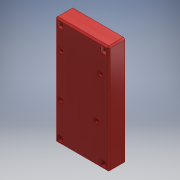
# Autodesk Inventor part: mangOH bottom
Saved by Autodesk Inventor 2017.3 (Build 213256000, 256)
## iProperties
Created: 2018-01-31
Part Number: mangOH bottom
Material: Generic
Document SubType Name: Modeling
Designer: michiel
Density: 1 g/cm^3
Appearance: Orange-Red
Author: michiel
Autodesk Inventor part; units mm, degrees
ref_plane "YZ Plane" through (0, 0, 0) normal (1, 0, 0) x (0, 1, 0)
ref_plane "XZ Plane" through (0, 0, 0) normal (0, 1, 0) x (-1, 0, 0)
ref_plane "XY Plane" through (0, 0, 0) normal (0, 0, 1) x (1, 0, 0)
sketch "Sketch1" plane through (0, 0, 0) normal (0, 1, 0) x (-1, 0, 0)
  line L0 (0, 0) -> (73, 0)
  line L1 (73, 0) -> (73, -148)
  line L2 (73, -148) -> (0, -148)
  line L3 (0, -148) -> (0, 0)
  dimension "d0" = 73
  dimension "d1" = 148
  constraints: 8 end point, 2 parallel, 1 horizontal, 1 perpendicular
  measures "d0" distance of L1.end L2.end
  measures "d1" distance of L0.end L1.end
extrude "Extrusion1" add sketch "Sketch1" against normal blind 4
sketch "Sketch2" plane through (0, 0, 0) normal (0, 1, 0) x (1, 0, 0)
  line L0 (-73, 148) -> (0, 148) projected
  line L1 (0, 148) -> (0, 0) projected
  line L2 (0, 148) -> (0, 0)
  line L3 (0, 0) -> (-73, 0) projected
  line L4 (0, 0) -> (-73, 0)
  line L5 (-73, 0) -> (-73, 148)
  line L6 (0, 148) -> (0, 144) construction
  line L7 (0, 148) -> (0, 0) construction
  line L8 (0, 144) -> (-4, 144) construction
  line L9 (-4, 144) -> (-69, 144)
  line L10 (-69, 144) -> (-69, 4)
  line L11 (-69, 4) -> (-4, 4)
  line L12 (-4, 4) -> (-4, 144)
  dimension "d4" = 4
  dimension "d5" = 4
  dimension "d6" = 90
  dimension "d7" = 65
  dimension "d8" = 140
  constraints: 18 end point, 3 perpendicular, 2 collinear, 2 horizontal, 1 point on line, 1 vertical
  measures "d4" distance of L0.end L6.end
  measures "d5" distance of L6.end L8.end
  measures "d6" angle of L6 L8
  measures "d7" distance of L8.end L9.end
  measures "d8" distance of L9.end L10.end
extrude "Extrusion2" add sketch "Sketch2" along normal blind 18
sketch "Sketch4" plane through (0, 0, 0) normal (0, 1, 0) x (1, 0, 0)
  line L0 (-4, 4) -> (-4, 144) projected
  line L1 (-4, 4) -> (-10, 4)
  line L2 (-10, 4) -> (-10, 10)
  line L3 (-10, 10) -> (-4, 10)
  line L4 (-4, 10) -> (-4, 4)
  point P0 (0, 0)
  dimension "d17" = 6
  dimension "d18" = 6
  constraints: 8 end point, 2 parallel, 1 horizontal, 1 perpendicular
  measures "d17" distance of L2.end L3.end
  measures "d18" distance of L1.end L2.end
extrude "Extrusion4" add sketch "Sketch4" along normal blind 15
sketch "Sketch9" plane through (0, -4, 0) normal (0, -1, 0) x (1, 0, 0)
  line L0 (0, 0) -> (0, -148) construction
  line L1 (0, 0) -> (-7, 0) construction
  line L2 (0, 0) -> (-73, 0) construction
  line L3 (-7, 0) -> (-7, -7) construction
  circle A0 centre (-7, -7) radius 2.05
  dimension "d60" = 7
  dimension "d61" = 7
  dimension "d62" = 4.1
  constraints: 4 end point, 1 centre point, 1 coincident, 1 perpendicular, 1 point on line
  measures "d60" distance of L0.start L1.end
  measures "d61" distance of L1.end L3.end
  measures "d62" diameter of A0
extrude "Extrusion10" cut sketch "Sketch9" against normal blind 20
sketch "Sketch10" plane through (0, -4, 0) normal (0, -1, 0) x (1, 0, 0)
  circle A0 centre (-7, -7) radius 2.05 construction
  line L0 (-7, -7) -> (-7, 0) construction
  line L1 (0, 0) -> (-73, 0) construction
  line L2 (-7, -7) -> (-10.6, -7) construction
  line L3 (-7, -7) -> (-3.4, -7) construction
  line L4 (-7, -7) -> (-7, -10.875) construction
  line L5 (-7, -7) -> (-7, -3.125) construction
  line L6 (-7, -3.125) -> (-10.6, -3.125)
  line L7 (-10.6, -3.125) -> (-10.6, -10.875)
  line L8 (-10.6, -10.875) -> (-3.4, -10.875)
  line L9 (-3.4, -10.875) -> (-3.4, -3.125)
  line L10 (-3.4, -3.125) -> (-7, -3.125)
  dimension "d65" = 3.6
  dimension "d66" = 3.6
  dimension "d67" = 3.875
  dimension "d68" = 3.875
  dimension "d69" = 7.75
  dimension "d70" = 7.2
  constraints: 20 end point, 4 perpendicular, 3 horizontal, 3 point on line, 2 vertical
  measures "d65" distance of L0.start L2.end
  measures "d66" distance of L0.start L3.end
  measures "d67" distance of L0.start L4.end
  measures "d68" distance of L0.start L5.end
  measures "d69" distance of L8.end L9.end
  measures "d70" distance of L7.end L8.end
extrude "Extrusion11" cut sketch "Sketch10" against normal blind 4
sketch "Sketch11" plane through (0, 0, 0) normal (0, 1, 0) x (1, 0, 0)
  line L0 (-10, 10) -> (-10, 4) projected
  line L1 (-10, 4) -> (-11.6, 4)
  line L2 (-69, 4) -> (-10, 4) projected
  line L3 (-11.6, 4) -> (-11.6, 11.6)
  line L4 (-11.6, 4) -> (-4, 4) construction
  line L5 (-11.6, 11.6) -> (-4, 11.6)
  line L6 (-4, 10.875) -> (-4, 144) projected
  line L7 (-4, 10) -> (-10, 10)
  line L8 (-10, 4) -> (-10, 10)
  line L9 (-10, 10) -> (-4, 10) projected
  line L10 (-4, 10) -> (-4, 11.6)
  point P0 (0, 0)
  dimension "d73" = 1.6
  dimension "d75" = 90
  dimension "d76" = 1.6
  constraints: 14 end point, 3 perpendicular, 2 point on line, 2 vertical, 1 collinear, 1 horizontal
  measures "d73" distance of L0.end L1.end
  measures "d75" angle of L4 L3
  measures "d76" distance between parallel lines of L5 L7
extrude "Extrusion12" add sketch "Sketch11" along normal blind 1.2
pattern_linear "Rectangular Pattern3" count 2 spacing 59 along (-1, 0, 0) count 2 spacing 134 along (0, 0, -1) of "Extrusion4", "Extrusion10", "Extrusion11"
sketch "Sketch12" plane through (0, 0, 0) normal (0, 1, 0) x (1, 0, 0)
  line L0 (-63, 4) -> (-10, 4) projected
  line L1 (-63, 4) -> (-61.4, 4)
  line L2 (-63, 4) -> (-63, 10) projected
  line L3 (-63, 4) -> (-63, 10)
  line L4 (-63, 10) -> (-69, 10)
  line L5 (-69, 10) -> (-69, 11.6)
  line L6 (-69, 11.6) -> (-61.4, 11.6)
  line L7 (-61.4, 11.6) -> (-61.4, 4)
  line L8 (-10, 144) -> (-63, 144) projected
  line L9 (-63, 144) -> (-61.4, 144)
  line L10 (-63, 138) -> (-63, 144) projected
  line L11 (-63, 144) -> (-63, 138)
  line L12 (-69, 138) -> (-63, 138) projected
  line L13 (-63, 138) -> (-69, 138)
  line L14 (-69, 138) -> (-69, 136.4)
  line L15 (-69, 137.125) -> (-69, 10.875) projected
  line L16 (-69, 136.4) -> (-61.4, 136.4)
  line L17 (-61.4, 136.4) -> (-61.4, 144)
  line L18 (-10, 144) -> (-10.6, 144) projected
  line L19 (-10, 144) -> (-11.6, 144)
  line L20 (-10, 144) -> (-8.4, 144) construction
  line L21 (-10, 144) -> (-10, 138) projected
  line L22 (-4, 138) -> (-10, 138) projected
  line L23 (-10, 144) -> (-10, 138)
  line L24 (-10, 138) -> (-4, 138)
  line L25 (-4, 138) -> (-4, 136.4)
  line L26 (-4, 10) -> (-4, 138) projected
  line L27 (-4, 136.4) -> (-11.6, 136.4)
  line L28 (-11.6, 136.4) -> (-11.6, 144)
  point P0 (0, 0)
  dimension "d85" = 1.6
  dimension "d86" = 1.6
  dimension "d87" = 90
  dimension "d88" = 1.6
  dimension "d89" = 1.6
  dimension "d90" = 90
  dimension "d91" = 1.6
  dimension "d92" = 180
  dimension "d93" = 1.6
  dimension "d94" = 90
  constraints: 38 end point, 8 perpendicular, 4 point on line, 2 collinear, 2 horizontal, 2 vertical
  measures "d85" distance of L0.start L1.end
  measures "d86" distance of L4.end L5.end
  measures "d87" angle of L4 L5
  measures "d88" distance of L8.end L9.end
  measures "d89" distance of L12.start L14.end
  measures "d90" angle of L16 L14
  measures "d91" distance of L8.start L19.end
  measures "d92" angle of L19 L20
  measures "d93" distance of L22.start L25.end
  measures "d94" angle of L25 L27
extrude "Extrusion13" add sketch "Sketch12" along normal blind 1.2
sketch "Sketch13" plane through (0, 0, 0) normal (0, 1, 0) x (1, 0, 0)
  line L0 (-4, 10) -> (-4, 138) construction
  line L1 (-4, 11.4955) -> (-4, 31.4955) construction
  line L2 (-4, 31.4955) -> (-8, 31.4955) construction
  line L3 (-8, 31.4955) -> (-69, 31.4955) construction
  line L4 (-69, 31.4955) -> (-69, 100.4955) construction
  line L5 (-69, 100.4955) -> (-8, 100.4955) construction
  line L6 (-8, 100.4955) -> (-8, 31.4955) construction
  line L7 (-69, 100.4955) -> (-69, 94.9955) construction
  line L8 (-69, 138) -> (-69, 10) construction
  line L9 (-69, 94.9955) -> (-16.5, 94.9955) construction
  circle A0 centre (-16.5, 94.9955) radius 3.5
  line L10 (-69, 94.9955) -> (-65.5, 94.9955) construction
  circle A1 centre (-65.5, 94.9955) radius 3.5
  line L11 (-65.5, 94.9955) -> (-2, 94.9955) construction
  line L12 (-65.5, 94.9955) -> (-65.5, 36.9955) construction
  circle A2 centre (-65.5, 36.9955) radius 3.5
  line L13 (-69, 31.4955) -> (-11.5, 31.4955) construction
  line L14 (-11.5, 31.4955) -> (-11.5, 36.9955) construction
  circle A3 centre (-11.5, 36.9955) radius 3.5
  circle A4 centre (-65.5, 36.9955) radius 1.55
  circle A5 centre (-16.5, 94.9955) radius 1.55
  circle A6 centre (-11.5, 36.9955) radius 1.55
  circle A7 centre (-65.5, 94.9955) radius 1.55
  point P0 (0, 0)
  dimension "d97" = 20
  dimension "d98" = 4
  dimension "d99" = 61
  dimension "d100" = 69
  dimension "d101" = 5.5
  dimension "d102" = 52.5
  dimension "d103" = 90
  dimension "d104" = 7
  dimension "d105" = 3.5
  dimension "d106" = 7
  dimension "d109" = 58
  dimension "d110" = 7
  dimension "d111" = 57.5
  dimension "d112" = 5.5
  dimension "d113" = 7
  dimension "d114" = 3.1
  dimension "d116" = 3.1
  dimension "d117" = 3.1
  dimension "d118" = 3.1
  constraints: 26 end point, 8 centre point, 8 coincident, 5 point on line, 3 horizontal, 3 perpendicular, 2 parallel, 1 vertical
  measures "d97" distance of L1.start L1.end
  measures "d98" distance of L1.end L2.end
  measures "d99" distance of L4.end L5.end
  measures "d100" distance of L3.end L4.end
  measures "d101" distance of L4.end L7.end
  measures "d102" distance of L7.end L9.end
  measures "d103" angle of L9 L7
  measures "d104" diameter of A0
  measures "d105" distance of L7.end L10.end
  measures "d106" diameter of A1
  measures "d109" distance of L11.start L12.end
  measures "d110" diameter of A2
  measures "d111" distance of L3.end L13.end
  measures "d112" distance of L13.end L14.end
  measures "d113" diameter of A3
  measures "d114" diameter of A4
  measures "d116" diameter of A5
  measures "d117" diameter of A6
  measures "d118" diameter of A7
extrude "Extrusion14" add sketch "Sketch13" along normal blind 15
sketch "Sketch14" plane through (-65.5, 0, -36.9955) normal (0, 1, 0) x (1, 0, 0)
  circle A0 centre (49, 58) radius 1.55 projected
  circle A1 centre (49, 58) radius 1.55
  circle A2 centre (0, 58) radius 1.55 projected
  circle A3 centre (0, 58) radius 1.55
  circle A4 centre (0, 0) radius 1.55
  circle A5 centre (54, 0) radius 1.55 projected
  circle A6 centre (54, 0) radius 1.55
  point P0 (65.5, -36.9955)
  dimension "d121" = 3.1
  constraints: 4 centre point, 3 coincident
  measures "d121" diameter of A6
extrude "Extrusion15" cut sketch "Sketch14" against normal blind 100
sketch "Sketch15" plane through (0, -4, 0) normal (0, -1, 0) x (1, 0, 0)
  circle A0 centre (-11.5, -36.9955) radius 1.55 construction
  line L0 (-11.5, -36.9955) -> (-11.5, -34.1955) construction
  line L1 (-11.5, -34.1955) -> (-14.6, -34.1955) construction
  line L2 (-14.6, -34.1955) -> (-14.6, -39.7955)
  line L3 (-14.6, -39.7955) -> (-8.4, -39.7955)
  line L4 (-14.6, -34.1955) -> (-8.4, -34.1955)
  line L5 (-8.4, -34.1955) -> (-8.4, -39.7955)
  circle A1 centre (-65.5, -36.9955) radius 1.55 construction
  line L6 (-65.5, -36.9955) -> (-62.4, -36.9955) construction
  line L7 (-62.4, -36.9955) -> (-62.4, -39.7955) construction
  line L8 (-62.4, -39.7955) -> (-68.6, -39.7955)
  line L9 (-68.6, -39.7955) -> (-68.6, -34.1955)
  line L10 (-68.6, -34.1955) -> (-62.4, -34.1955)
  line L11 (-62.4, -34.1955) -> (-62.4, -39.7955)
  circle A2 centre (-16.5, -94.9955) radius 1.55 construction
  line L12 (-16.5, -94.9955) -> (-16.5, -97.7955) construction
  line L13 (-16.5, -97.7955) -> (-13.4, -97.7955) construction
  line L14 (-13.4, -97.7955) -> (-19.6, -97.7955)
  line L15 (-19.6, -97.7955) -> (-19.6, -92.1955)
  line L16 (-19.6, -92.1955) -> (-13.4, -92.1955)
  line L17 (-13.4, -92.1955) -> (-13.4, -97.7955)
  line L18 (-65.5, -94.9955) -> (-65.5, -97.7955) construction
  line L19 (-65.5, -97.7955) -> (-62.4, -97.7955) construction
  line L20 (-62.4, -97.7955) -> (-68.6, -97.7955)
  line L21 (-68.6, -97.7955) -> (-68.6, -92.1955)
  line L22 (-68.6, -92.1955) -> (-62.4, -92.1955)
  line L23 (-62.4, -92.1955) -> (-62.4, -97.7955)
  point P0 (0, 0)
  dimension "d124" = 2.8
  dimension "d125" = 3.1
  dimension "d126" = 5.6
  dimension "d127" = 6.2
  dimension "d130" = 3.1
  dimension "d131" = 2.8
  dimension "d132" = 6.2
  dimension "d133" = 5.6
  dimension "d134" = 2.8
  dimension "d135" = 3.1
  dimension "d136" = 6.2
  dimension "d137" = 5.6
  dimension "d138" = 2.8
  dimension "d139" = 3.1
  dimension "d140" = 6.2
  dimension "d141" = 5.6
  constraints: 48 end point, 8 perpendicular, 6 horizontal, 6 parallel, 4 vertical
  measures "d124" distance of L0.start L0.end
  measures "d125" distance of L0.end L1.end
  measures "d126" distance of L1.end L2.end
  measures "d127" distance of L2.end L3.end
  measures "d130" distance of L6.start L6.end
  measures "d131" distance of L6.end L7.end
  measures "d132" distance of L9.end L10.end
  measures "d133" distance of L8.end L9.end
  measures "d134" distance of L12.start L12.end
  measures "d135" distance of L12.end L13.end
  measures "d136" distance of L15.end L16.end
  measures "d137" distance of L14.end L15.end
  measures "d138" distance of L18.start L18.end
  measures "d139" distance of L18.end L19.end
  measures "d140" distance of L21.end L22.end
  measures "d141" distance of L20.end L21.end
extrude "Extrusion17" cut sketch "Sketch15" against normal blind 3
sketch "Sketch17" plane through (0, 18, 0) normal (0, 1, 0) x (1, 0, 0)
  line L0 (-69, 4) -> (-69, 144) projected
  line L1 (-4, 144) -> (-4, 4) projected
  line L2 (-69, 144) -> (-4, 144)
  line L3 (-4, 144) -> (-4, 4)
  line L4 (-4, 4) -> (-69, 4)
  line L5 (-69, 4) -> (-69, 144)
  line L6 (-4, 4) -> (-5.9, 4) construction
  line L7 (-5.9, 4) -> (-5.9, 2.1828) construction
  line L8 (-5.9, 2.1828) -> (-4, 2.1828) construction
  line L9 (-4, 2.1828) -> (-4, 4) construction
  line L10 (-4, 4) -> (-1.9, 4) construction
  line L11 (-1.9, 4) -> (-1.9, 1.9) construction
  line L12 (-69, 144) -> (-71.1, 144) construction
  line L13 (-71.1, 144) -> (-71.1, 146.1) construction
  line L14 (-71.1, 146.1) -> (-1.9, 146.1)
  line L15 (-1.9, 146.1) -> (-1.9, 1.9)
  line L16 (-1.9, 1.9) -> (-71.1, 1.9)
  line L17 (-71.1, 1.9) -> (-71.1, 146.1)
  point P0 (0, 0)
  dimension "d144" = 1.9
  dimension "d145" = 2.1
  dimension "d146" = 2.1
  dimension "d147" = 2.1
  dimension "d148" = 2.1
  constraints: 32 end point, 6 parallel, 6 perpendicular, 4 horizontal
  measures "d144" distance of L8.end L7.end
  measures "d145" distance of L1.end L10.end
  measures "d146" distance of L10.end L11.end
  measures "d147" distance of L0.end L12.end
  measures "d148" distance of L12.end L13.end
extrude "Extrusion18" cut sketch "Sketch17" against normal blind 4
chamfer "Chamfer1" distance 2 angle 45 8 edges at (-36.5, -4, 0) (-73, 7, 0) (-73, -4, -74) (0, 7, 0) (0, -4, -74) (0, 7, -148) (-36.5, -4, -148) (-73, 7, -148)
body "Solid1"
